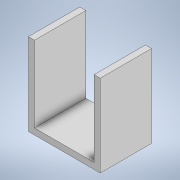
# Autodesk Inventor part: armj1
Saved by Autodesk Inventor 2020 (Build 240168000, 168)
## iProperties
Created: 2021-03-31
Part Number: armj1
Material: Generic
Document SubType Name: Modeling
Designer: super
Density: 1 g/cm^3
Appearance: Default
Author: super
Autodesk Inventor part; units mm, degrees
ref_plane "YZ Plane" through (0, 0, 0) normal (1, 0, 0) x (0, 1, 0)
ref_plane "XZ Plane" through (0, 0, 0) normal (0, 1, 0) x (-1, 0, 0)
ref_plane "XY Plane" through (0, 0, 0) normal (0, 0, 1) x (1, 0, 0)
sketch "Sketch1" plane through (0, 0, 0) normal (0, 0, 1) x (1, 0, 0)
  line L0 (0, 80) -> (0, 0)
  line L1 (0, 0) -> (70, 0)
  line L2 (70, 0) -> (70, 80)
  line L3 (6, 80) -> (6, 6)
  line L4 (6, 6) -> (64, 6)
  line L5 (64, 6) -> (64, 80)
  line L6 (0, 80) -> (6, 80)
  line L7 (64, 80) -> (70, 80)
  dimension "d0" = 70
  dimension "d1" = 80
  dimension "d2" = 80
  dimension "d3" = 6
  constraints: 16 end point, 3 perpendicular, 2 horizontal, 1 vertical, 2 other
  measures "d0" distance of L0.end L1.end
  measures "d1" distance of L1.end L2.end
  measures "d2" distance of L0.start L0.end
  measures "d3" distance between parallel lines of L0 L3
extrude "Extrusion1" add sketch "Sketch1" along normal blind 50
body "Solid1"
